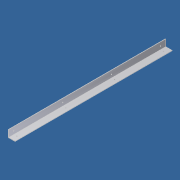
# Autodesk Inventor part: GE-12063
Saved by Autodesk Inventor 2012 (Build 160160000, 160)
## iProperties
Created: 2011-10-29
Part Number: GE-12063
Document SubType Name: Modeling
Designer: dfoster
Density: 1 g/cm^3
Description: Angle, Ball Ramp
Material: Default
Title: Angle, Ball Ramp
Author: dfoster
Autodesk Inventor part; units mm, degrees
ref_plane "YZ Plane" through (0, 0, 0) normal (1, 0, 0) x (0, 1, 0)
ref_plane "XZ Plane" through (0, 0, 0) normal (0, 1, 0) x (-1, 0, 0)
ref_plane "XY Plane" through (0, 0, 0) normal (0, 0, 1) x (1, 0, 0)
sketch "Sketch1" plane through (0, 0, 0) normal (0, 0, 1) x (1, 0, 0)
  line L0 (0, 0) -> (0, 50.8)
  line L1 (0, 50.8) -> (3.175, 50.8)
  line L2 (3.175, 50.8) -> (3.175, 3.175)
  line L3 (3.175, 3.175) -> (50.8, 3.175)
  line L4 (50.8, 3.175) -> (50.8, 0)
  line L5 (50.8, 0) -> (0, 0)
  dimension "d0" = 50.8
  dimension "d1" = 3.175
  dimension "d4" = 50.8
  constraints: 12 end point, 4 parallel, 3 perpendicular, 1 vertical
  measures "d0" distance of L4.end L0.start
  measures "d1" distance between parallel lines of L3 L5
  measures "d4" distance of L0.start L0.end
extrude "Extrusion1" add sketch "Sketch1" along normal blind 1143
hole "Hole1" at (25.4, 3.175, 1104.9) direction (0, -1, 0) diameter 6.731 depth 25.4 tip angle 118
pattern_linear "Rectangular Pattern1" count 4 spacing 355.6 along (0, 0, -1) of "Hole1"
hole "Hole2" at (3.175, 25.4, 1104.9) direction (-1, 0, 0) diameter 6.731 depth 25.4 tip angle 118
pattern_linear "Rectangular Pattern2" count 4 spacing 355.6 along (0, 0, -1) of "Hole2", "Hole1"
body "Solid1"
